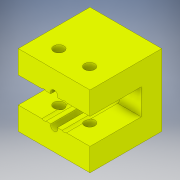
# Autodesk Inventor part: sevo_piece
Saved by Autodesk Inventor 2019 (Build 230136000, 136)
## iProperties
Created: 2019-02-02
Part Number: sevo_piece
Material: Generic
Document SubType Name: Modeling
Designer: suchanek
Density: 1 g/cm^3
Appearance: Default
Author: suchanek
Autodesk Inventor part; units mm, degrees
ref_plane "YZ Plane" through (0, 0, 0) normal (1, 0, 0) x (0, 1, 0)
ref_plane "XZ Plane" through (0, 0, 0) normal (0, 1, 0) x (-1, 0, 0)
ref_plane "XY Plane" through (0, 0, 0) normal (0, 0, 1) x (1, 0, 0)
sketch "Sketch1" plane through (0, 0, 0) normal (0, 0, 1) x (1, 0, 0)
  circle A0 centre (0, 0) radius 10
  circle A1 centre (0, 7) radius 0.85
  circle A2 centre (-4.9497, 4.9497) radius 0.85
  circle A3 centre (-7, 0) radius 0.85
  circle A4 centre (-4.9497, -4.9497) radius 0.85
  circle A5 centre (0, -7) radius 0.85
  circle A6 centre (4.9497, -4.9497) radius 0.85
  circle A7 centre (7, 0) radius 0.85
  circle A8 centre (4.9497, 4.9497) radius 0.85
  dimension "d0" = 20
  dimension "d1" = 7
  dimension "d2" = 1.7
  dimension "d5" = 360
  constraints: 9 centre point, 2 coincident, 1 vertical alignment, 17 other
  measures "d0" diameter of A0
  measures "d1" distance of A1.centre point (0, 0)
  measures "d2" diameter of A1
extrude "Extrusion1" add sketch "Sketch1" along normal blind 10
sketch "Sketch2" plane through (0, 0, 10) normal (0, 0, 1) x (1, 0, 0)
  line L0 (17.5, -17.5) -> (-17.5, -17.5)
  line L1 (-17.5, -17.5) -> (-17.5, 17.5)
  line L2 (-17.5, 17.5) -> (17.5, 17.5)
  line L3 (17.5, 17.5) -> (17.5, -17.5)
  line L4 (17.5, -17.5) -> (-17.5, 17.5) construction
  line L5 (-17.5, -17.5) -> (17.5, 17.5) construction
  point P0 (0, 0)
  dimension "d9" = 35
  dimension "d10" = 35
  constraints: 12 end point, 2 midpoint, 2 parallel, 1 horizontal, 1 perpendicular
  measures "d9" distance of L1.end L2.end
  measures "d10" distance of L0.end L1.end
extrude "Extrusion2" add sketch "Sketch2" against normal blind 10
sketch "Sketch3" plane through (0, 0, 10) normal (0, 0, 1) x (1, 0, 0)
  line L0 (17.5, 17.5) -> (17.5, -17.5) projected
  line L1 (-17.5, -17.5) -> (17.5, -17.5)
  line L2 (17.5, -17.5) -> (17.5, -6.35)
  line L3 (17.5, -6.35) -> (-17.5, -6.35)
  line L4 (-17.5, -6.35) -> (-17.5, -17.5)
  line L5 (-17.5, -17.5) -> (-17.5, 17.5) projected
  line L6 (17.5, 17.5) -> (-17.5, 17.5)
  line L7 (-17.5, 17.5) -> (-17.5, 6.35)
  line L8 (-17.5, 6.35) -> (17.5, 6.35)
  line L9 (17.5, 6.35) -> (17.5, 17.5)
  line L10 (0, 0) -> (4.0758, 0)
  dimension "d36" = 12.7
  constraints: 18 end point, 4 parallel, 3 horizontal, 2 perpendicular, 2 point on line, 1 other
  measures "d36" distance between parallel lines of L8 L3
extrude "Extrusion3" add sketch "Sketch3" along normal blind 25 contours L0 L8 L5 L6 | L0 L1 L4 L3
sketch "Sketch4" plane through (0, 0, 10) normal (0, 0, 1) x (1, 0, 0)
  point P0 (0, 0)
  point P1 (7, 0)
  point P2 (4.9497, 4.9497)
  point P3 (0, 7)
  point P4 (-4.9497, 4.9497)
  point P5 (-7, 0)
  point P6 (-4.9497, -4.9497)
  point P7 (0, -7)
  point P8 (4.9497, -4.9497)
  dimension "d17" = 7
  dimension "d20" = 360
  constraints: 1 horizontal alignment, 9 other
  measures "d17" distance of point (0, 0) point (7, 0)
hole "Hole1" at (0, -7, 10) at (-4.9497, -4.9497, 10) at (-7, 0, 10) at (4.9497, -4.9497, 10) at (4.9497, 4.9497, 10) at (7, 0, 10) at (-4.9497, 4.9497, 10) at (0, 7, 10) direction (0, 0, -1) diameter 1.8 depth 10 start extended yes counterbore diameter 3.5 counterbore depth 2
sketch "Sketch5" plane through (-17.5, 17.5, 0) normal (0, 1, 0) x (1, 0, 0)
  circle A0 centre (10, -25.2) radius 2.5
  circle A1 centre (25, -25.2) radius 2.5
  line L0 (17.5, 0) -> (17.5, -18.6414)
  line L1 (0, -35) -> (0, 0) projected
  line L2 (0, 0) -> (35, 0) projected
  line L3 (11.5006, -10) -> (0, -10) projected
  dimension "d29" = 5
  dimension "d30" = 5
  dimension "d32" = 15
  dimension "d37" = 15.2
  constraints: 2 centre point, 2 end point, 1 horizontal alignment, 1 symmetric about line, 1 vertical
  measures "d29" diameter of A0
  measures "d30" diameter of A1
  measures "d32" distance of A1.centre A0.centre
  measures "d37" distance from line of L3 A0.centre
extrude "Extrusion4" cut sketch "Sketch5" against normal through all
body "Solid1"
